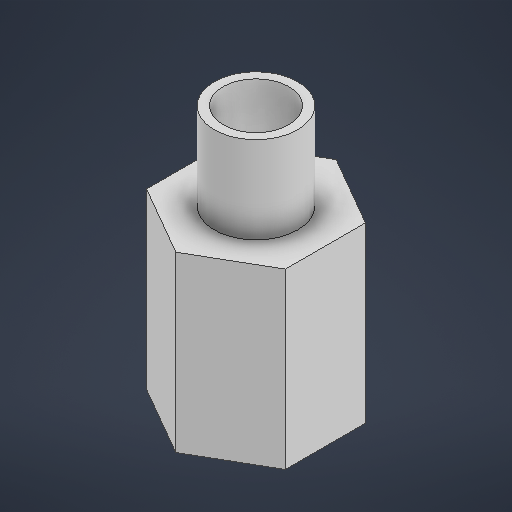
# Autodesk Inventor part: expansor de conexion
Saved by Autodesk Inventor 2026.1 (Build 301233000, 233)
## iProperties
Created: 2025-12-08
Part Number: expansor de conexion
Material: Genérico
Document SubType Name: Modeling
Designer: vickh
Density: 1 g/cm^3
Appearance: Valor por defecto
Author: vickh
Autodesk Inventor part; units mm, degrees
ref_plane "YZ Plane" through (0, 0, 0) normal (1, 0, 0) x (0, 1, 0)
ref_plane "XZ Plane" through (0, 0, 0) normal (0, 1, 0) x (-1, 0, 0)
ref_plane "XY Plane" through (0, 0, 0) normal (0, 0, 1) x (1, 0, 0)
sketch "Boceto1" plane through (0, 0, 0) normal (0, 1, 0) x (-1, 0, 0)
  line L0 (0, 4.6188) -> (4, 2.3094)
  line L1 (4, 2.3094) -> (4, -2.3094)
  line L2 (4, -2.3094) -> (0, -4.6188)
  line L3 (0, -4.6188) -> (-4, -2.3094)
  line L4 (-4, -2.3094) -> (-4, 2.3094)
  line L5 (-4, 2.3094) -> (0, 4.6188)
  circle A0 centre (0, 0) radius 1.9
  point P0 (4, 0)
  dimension "d0" = 3.8
  dimension "d2" = 4
  constraints: 12 end point, 2 coincident, 1 centre point, 1 midpoint, 1 vertical, 13 other
  measures "d0" diameter of A0
  measures "d2" distance of point (4, 0) point (0, 0)
extrude "Extrusión1" add sketch "Boceto1" along normal mid plane 10
sketch "Boceto2" plane through (0, 5, 0) normal (0, 1, 0) x (1, 0, 0)
  circle A0 centre (0, 0) radius 1.9 projected
  circle A1 centre (0, 0) radius 2.4
  dimension "d5" = 4.8
  constraints: 1 centre point, 1 coincident
  measures "d5" diameter of A1
extrude "Extrusión2" add sketch "Boceto2" along normal blind 5
